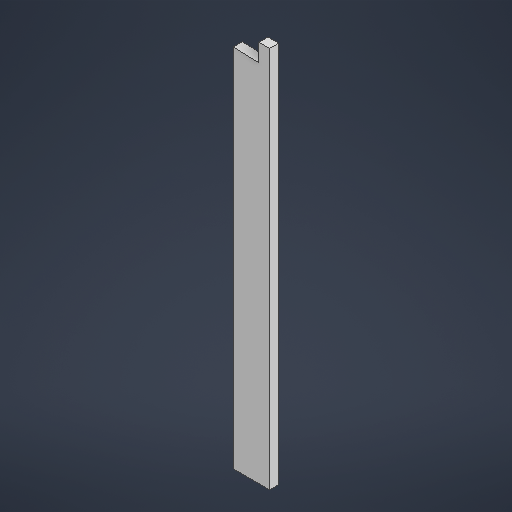
# Autodesk Inventor part: protostand2
Saved by Autodesk Inventor 2026.2 (Build 302298000, 298)
## iProperties
Created: 2026-04-18
Part Number: protostand2
Material: Generic
Document SubType Name: Modeling
Designer: danda
Density: 1 g/cm^3
Appearance: Default
Author: danda
Autodesk Inventor part; units mm, degrees
ref_plane "YZ Plane" through (0, 0, 0) normal (1, 0, 0) x (0, 1, 0)
ref_plane "XZ Plane" through (0, 0, 0) normal (0, 1, 0) x (-1, 0, 0)
ref_plane "XY Plane" through (0, 0, 0) normal (0, 0, 1) x (1, 0, 0)
sketch "Sketch1" plane through (0, 0, 0) normal (0, 0, 1) x (1, 0, 0)
  line L0 (27.6851, 142.7138) -> (33.5851, 142.7138)
  line L1 (33.5851, 142.7138) -> (33.5851, 132.7138)
  line L2 (33.5851, 132.7138) -> (27.6851, 132.7138)
  line L3 (27.6851, 132.7138) -> (27.6851, 142.7138)
  line L4 (33.5851, 132.7138) -> (33.5851, -67.2862)
  line L5 (33.5851, -67.2862) -> (13.5851, -67.2862)
  line L6 (13.5851, -67.2862) -> (13.5851, 133.4123)
  line L7 (33.5851, 132.7138) -> (13.5851, 133.4123)
  line L8 (33.5851, 132.7138) -> (53.5973, 132.7138) construction
  point P0 (0, 0)
  point P1 (27.6851, 132.9199)
  dimension "d0" = 5.9
  dimension "d1" = 10
  dimension "d2" = 200
  dimension "d3" = 20
  dimension "d4" = 178
  constraints: 18 end point, 5 perpendicular, 2 horizontal, 1 equal length, 1 point on line
  measures "d0" distance of L0.start L0.end
  measures "d1" distance of L0.end L1.end
  measures "d2" distance of L1.end L4.end
  measures "d3" distance of L4.end L5.end
  measures "d4" angle of L8 L7
extrude "Extrusion1" add sketch "Sketch1" along normal blind 5
body "Solid1"
